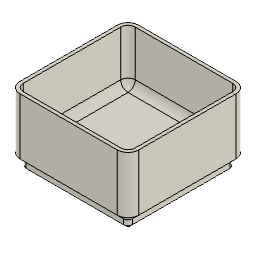
Discard Tray Gridfinity 1x1 z=3.5 (Autodesk Fusion 360 design; units mm, degrees)
Autodesk Fusion 360 part; units mm, degrees
ref_plane "WorkPlane1" through (0, 0, 0) normal (0, 0, 1) x (1, 0, 0) in component "Gridfinity bin 1x1x3"
sketch "Base plate sketch" plane through (0, 0, 0) normal (0, 0, 1) x (1, 0, 0) in component "Gridfinity bin 1x1x3"
  line L0 (-0.25, -0.25) -> (41.75, -0.25)
  line L1 (41.75, -0.25) -> (41.75, 41.75)
  line L2 (41.75, 41.75) -> (-0.25, 41.75)
  line L3 (-0.25, 41.75) -> (-0.25, -0.25)
  dimension "d2" = 0.25
  dimension "d3" = 0.25
  dimension "d4" = 42
  dimension "d5" = 42
  constraint horizontal L0
  constraint vertical L1
  constraint horizontal L2
  constraint vertical L3
  measures "d2" vertical distance of origin L0.start
  measures "d3" horizontal distance of origin L2.end
  measures "d4" horizontal distance of L0.start L0.end
  measures "d5" vertical distance of L0.end L1.end
extrude "Base top section extrude" add sketch "Base plate sketch" against normal blind 2.4 makes body 1 in component "Gridfinity bin 1x1x3"
fillet "Base corner fillet" radius 4 8 edges at (-0.25, -0.25, -1.2) (41.75, -0.25, -1.2) (41.75, -0.25, -1.2) (41.75, 41.75, -1.2) (41.75, 41.75, -1.2) (-0.25, 41.75, -1.2) (-0.25, 41.75, -1.2) (-0.25, -0.25, -1.2) on bodies 1 in component "Gridfinity bin 1x1x3"
chamfer "Chamfer1" distance 2.4 angle 45 8 edges at (0.9216, 40.5784, -2.4) (-0.25, 20.75, -2.4) (0.9216, 0.9216, -2.4) (20.75, -0.25, -2.4) (40.5784, 0.9216, -2.4) (41.75, 20.75, -2.4) (40.5784, 40.5784, -2.4) (20.75, 41.75, -2.4) on bodies 1 in component "Gridfinity bin 1x1x3"
extrude "Extrude2" add 1 faces at (15.6168, 15.0833, -2.4) along direction (0, 0, -1) blind 2.6 on bodies 1 bodies 1 in component "Gridfinity bin 1x1x3"
chamfer "Chamfer2" distance 0.8 angle 45 8 edges at (2.6186, 38.8814, -5) (20.75, 39.35, -5) (38.8814, 38.8814, -5) (39.35, 20.75, -5) (38.8814, 2.6186, -5) (20.75, 2.15, -5) (2.6186, 2.6186, -5) (2.15, 20.75, -5) on bodies 1 in component "Gridfinity bin 1x1x3"
pattern_linear "R-Pattern1" count 1 spacing 42 along (1, 0, 0) of bodies 1 merged in component "Gridfinity bin 1x1x3"
sketch "Simple box sketch" plane through (0, 0, 0) normal (0, 0, 1) x (1, 0, 0) in component "Gridfinity bin 1x1x3"
  line L0 (0, 0) -> (41.5, 0)
  line L1 (41.5, 0) -> (41.5, 41.5)
  line L2 (41.5, 41.5) -> (0, 41.5)
  line L3 (0, 41.5) -> (0, 0)
  dimension "d18" = 41.5
  dimension "d19" = 41.5
  constraint horizontal L0
  constraint vertical L1
  constraint horizontal L2
  constraint vertical L3
  constraint coincident L0.start L3
  constraint coincident L3.end L0
  measures "d18" horizontal distance of L0.start L0.end
  measures "d19" vertical distance of L0.end L1.end
extrude "Simple box extrude" add sketch "Simple box sketch" along normal blind 19.5 separate body makes body 2 in component "Gridfinity bin 1x1x3"
fillet "Bin body corner fillets" radius 3.75 8 edges at (0, 41.5, 9.75) (41.5, 41.5, 9.75) (41.5, 0, 9.75) (0, 0, 9.75) (0, 0, 9.75) (0, 41.5, 9.75) (41.5, 41.5, 9.75) (41.5, 0, 9.75) on bodies 2 in component "Gridfinity bin 1x1x3"
ref_plane "WorkPlane2" through (0, 0, 19.5) normal (0, 0, 1) x (1, 0, 0) in component "Gridfinity bin 1x1x3"
sketch "Inner cutout sketch" plane through (0, 0, 19.5) normal (0, 0, 1) x (1, 0, 0) in component "Gridfinity bin 1x1x3"
  line L0 (1.2, 1.2) -> (40.3, 1.2)
  line L1 (40.3, 1.2) -> (40.3, 40.3)
  line L2 (40.3, 40.3) -> (1.2, 40.3)
  line L3 (1.2, 40.3) -> (1.2, 1.2)
  dimension "d25" = 1.2
  dimension "d26" = 1.2
  dimension "d27" = 39.1
  dimension "d28" = 39.1
  constraint horizontal L0
  constraint vertical L1
  constraint horizontal L2
  constraint vertical L3
  measures "d25" vertical distance of origin L0.start
  measures "d26" horizontal distance of origin L2.end
  measures "d27" horizontal distance of L0.start L0.end
  measures "d28" vertical distance of L0.end L1.end
extrude "Inner cutout extrude" add sketch "Inner cutout sketch" against normal blind 18.5 separate body makes body 3 in component "Gridfinity bin 1x1x3"
fillet "Fillet3" radius 2.55 8 edges at (1.2, 1.2, 10.25) (40.3, 1.2, 10.25) (40.3, 1.2, 10.25) (40.3, 40.3, 10.25) (40.3, 40.3, 10.25) (1.2, 40.3, 10.25) (1.2, 40.3, 10.25) (1.2, 1.2, 10.25) on bodies 3 in component "Gridfinity bin 1x1x3"
fillet "Fillet4" radius 2.55 8 edges at (20.75, 40.3, 1) (39.5531, 39.5531, 1) (40.3, 20.75, 1) (39.5531, 1.9469, 1) (20.75, 1.2, 1) (1.9469, 1.9469, 1) (1.2, 20.75, 1) (1.9469, 39.5531, 1) on bodies 3 in component "Gridfinity bin 1x1x3"
combine "Combine1" operation cut target body 2 tool bodies 3 in component "Gridfinity bin 1x1x3"
ref_plane "WorkPlane3" through (0, 0, 0) normal (0, 0, 1) x (1, 0, 0) in component "Gridfinity bin 1x1x3"
sketch "Base clearance cut sketch" plane through (0, 0, 0) normal (0, 0, 1) x (1, 0, 0) in component "Gridfinity bin 1x1x3"
  line L0 (3.75, 0) -> (37.75, 0)
  line L1 (41.5, 3.75) -> (41.5, 37.75)
  line L2 (37.75, 41.5) -> (3.75, 41.5)
  line L3 (0, 37.75) -> (0, 3.75)
  arc A0 (37.75, 0) -> (41.5, 3.75) centre (37.75, 3.75) ccw
  arc A1 (41.5, 37.75) -> (37.75, 41.5) centre (37.75, 37.75) ccw
  arc A2 (3.75, 41.5) -> (0, 37.75) centre (3.75, 37.75) ccw
  arc A3 (0, 3.75) -> (3.75, 0) centre (3.75, 3.75) ccw
  arc A4 (37.75, -10) -> (51.5, 3.75) centre (37.75, 3.75) ccw
  line L4 (51.5, 3.75) -> (51.5, 37.75)
  arc A5 (51.5, 37.75) -> (37.75, 51.5) centre (37.75, 37.75) ccw
  line L5 (37.75, 51.5) -> (3.75, 51.5)
  arc A6 (3.75, 51.5) -> (-10, 37.75) centre (3.75, 37.75) ccw
  line L6 (-10, 37.75) -> (-10, 3.75)
  arc A7 (-10, 3.75) -> (3.75, -10) centre (3.75, 3.75) ccw
  line L7 (3.75, -10) -> (37.75, -10)
  point P0 (41.5, 0)
  point P1 (41.5, 41.5)
  dimension "d36" = 41.5
  dimension "d37" = 41.5
  dimension "d38" = 3.75
  dimension "d39" = 10
  constraint horizontal L0
  constraint vertical L1
  constraint horizontal L2
  constraint vertical L3
  constraint coincident origin L3
  constraint coincident origin L0
  constraint coincident P0 L0
  constraint coincident P0 L1
  constraint tangent L0 A0
  constraint tangent L1 A0
  constraint coincident P1 L1
  constraint coincident P1 L2
  constraint tangent L1 A1
  constraint tangent L2 A1
  constraint tangent L2 A2
  constraint tangent L3 A2
  constraint tangent L3 A3
  constraint tangent L0 A3
  constraint equal A0 A1
  constraint equal A1 A2
  constraint equal A2 A3
  measures "d36" horizontal distance of origin P0
  measures "d37" vertical distance of P0 P1
  measures "d38" radius of A0
extrude "Base side clearance cut" cut sketch "Base clearance cut sketch" along normal blind 1000 and the other way blind 1000 bodies 1 2 in component "Gridfinity bin 1x1x3"
combine "Combine2" operation add target body 2 tool bodies 1 1 in component "Gridfinity bin 1x1x3"
component "Gridfinity bin 1x1x3" placed x (1, 0, 0) y (0, 1, 0) z (0, 0, 1) at (0, 0, 0)
equation "d6 = -( 2.40 mm )"
equation "d29 = -( 18.50 mm )"
named bodies: "Base", "Gridfinity bin 1x1x3", "Inner cutout"
